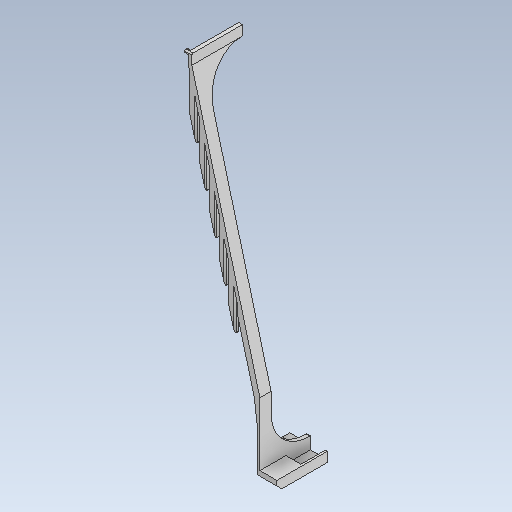
# Autodesk Inventor part: Держатель каскада
Saved by Autodesk Inventor 2020 (Build 240168000, 168)
## iProperties
Created: 2021-05-17
Part Number: Держатель каскада
Material: Типовые
Document SubType Name: Modeling
Designer: I_Love_U_Bogdan
Density: 1 g/cm^3
Appearance: По умолчанию
Author: I_Love_U_Bogdan
Autodesk Inventor part; units mm, degrees
ref_plane "YZ Plane" through (0, 0, 0) normal (1, 0, 0) x (0, 1, 0)
ref_plane "XZ Plane" through (0, 0, 0) normal (0, 1, 0) x (-1, 0, 0)
ref_plane "XY Plane" through (0, 0, 0) normal (0, 0, 1) x (1, 0, 0)
sketch "Эскиз1" plane through (0, 0, 0) normal (0, 0, 1) x (1, 0, 0)
  line L0 (-10.5496, 43.8447) -> (-9.5496, 40.1126)
  line L1 (-9.5496, 26.5897) -> (-9.5496, 40.1126)
  line L2 (-9.5496, 26.5897) -> (-10.5496, 30.3217)
  line L3 (-10.5496, 30.3217) -> (-10.5496, 43.8447)
  line L4 (-6.5496, 28.9165) -> (-5.5496, 25.1844)
  line L5 (-5.5496, 11.6615) -> (-5.5496, 25.1844)
  line L6 (-5.5496, 11.6615) -> (-6.5496, 15.3935)
  line L7 (-6.5496, 15.3935) -> (-6.5496, 28.9165)
  line L8 (-14.5496, 58.7729) -> (-13.5496, 55.0408)
  line L9 (-13.5496, 41.5179) -> (-13.5496, 55.0408)
  line L10 (-13.5496, 41.5179) -> (-14.5496, 45.2499)
  line L11 (-14.5496, 45.2499) -> (-14.5496, 58.7729)
  line L12 (-18.5496, 73.7011) -> (-17.5496, 69.969)
  line L13 (-17.5496, 56.4461) -> (-17.5496, 69.969)
  line L14 (-17.5496, 56.4461) -> (-18.5496, 60.1781)
  line L15 (-18.5496, 60.1781) -> (-18.5496, 73.7011)
  line L16 (-22.5496, 88.6293) -> (-21.5496, 84.8972)
  line L17 (-21.5496, 71.3743) -> (-21.5496, 84.8972)
  line L18 (-21.5496, 71.3743) -> (-22.5496, 75.1063)
  line L19 (-22.5496, 75.1063) -> (-22.5496, 88.6293)
  line L20 (-26.5496, 103.5575) -> (-25.5496, 99.8254)
  line L21 (-25.5496, 86.3025) -> (-25.5496, 99.8254)
  line L22 (-25.5496, 86.3025) -> (-26.5496, 90.0345)
  line L23 (-26.5496, 90.0345) -> (-26.5496, 103.5575)
  line L24 (-5.5496, 31.614) -> (-25.7752, 107.0972)
  line L25 (-25.7752, 110.0635) -> (-25.7752, 107.0972)
  line L26 (-5.5496, 25.1844) -> (-5.5496, 31.614)
  line L27 (-6.5496, 28.9165) -> (-6.5496, 36.5052)
  line L28 (-9.5496, 40.1126) -> (-9.5496, 47.7014)
  line L29 (-10.5496, 43.8447) -> (-10.5496, 51.4334)
  line L30 (-13.5496, 55.0408) -> (-13.5496, 62.6296)
  line L31 (-14.5496, 58.7729) -> (-14.5496, 66.3616)
  line L32 (-17.5496, 69.969) -> (-17.5496, 77.5578)
  line L33 (-18.5496, 73.7011) -> (-18.5496, 81.2898)
  line L34 (-25.5496, 99.8254) -> (-25.5496, 106.2551)
  line L35 (-26.5496, 103.5575) -> (-26.5496, 108.8932)
  line L36 (-21.5496, 84.8972) -> (-21.5496, 91.3269)
  line L37 (-22.5496, 88.6293) -> (-22.5496, 96.218)
  line L38 (-5.5496, 32.7732) -> (-25.7752, 108.2563)
  line L39 (-5.5496, 31.614) -> (-5.5496, 32.7732)
  line L40 (-25.5496, 106.2551) -> (-25.5496, 107.4142)
  line L41 (-21.5496, 84.8972) -> (-21.5496, 92.486)
  line L42 (-5.5496, 17.457) -> (-26.5496, 95.8301)
  line L43 (-28.0432, 111.0635) -> (-27.7752, 110.0635)
  line L44 (-27.7752, 110.0635) -> (-25.7752, 110.0635)
  line L45 (-25.7752, 110.0635) -> (-25.7752, 111.0635)
  line L46 (-25.7752, 111.0635) -> (-28.0432, 111.0635)
  line L47 (-29.7344, 117.3754) -> (-25.7752, 117.3754)
  line L48 (-28.0432, 111.0635) -> (-29.7344, 117.3754)
  line L49 (-25.7752, 111.0635) -> (-28.0432, 111.0635)
  line L50 (-25.7752, 117.3754) -> (-25.7752, 111.0635)
  line L51 (-25.7752, 111.0635) -> (-27.2752, 111.0635)
  line L52 (-27.2752, 111.0635) -> (-27.2752, 112.5635)
  line L53 (-27.2752, 112.5635) -> (-25.7752, 112.5635)
  line L54 (-25.7752, 112.5635) -> (-25.7752, 111.0635)
  line L55 (-25.7752, 112.5635) -> (-24.2752, 112.5635)
  line L56 (-24.2752, 112.5635) -> (-24.2752, 108.4538)
  line L57 (-30.0024, 118.3754) -> (0.8622, 3.1871)
  line L58 (-30.9752, 118.3754) -> (-30.0024, 118.3754)
  line L59 (-30.9752, 108.4603) -> (-30.9752, 118.3754)
  line L60 (-30.4811, 104.7073) -> (-30.9752, 108.4603)
  line L61 (-3.5492, 4.1961) -> (-30.4811, 104.7073)
  line L62 (-3.5492, 4.1961) -> (-3.5492, -15.1653)
  spline S0 degree 3 poles (-3.5492, -15.1653) (-3.5492, -15.4959) (-3.5491, -15.8265) (-3.5502, -16.4901) (-3.5515, -16.823) (-3.5561, -17.1584) knots 0 0 0 0 0.5 0.5 1 1 1 1 weights 1 1 1 1 1 1
  line L63 (-3.5561, -17.1584) -> (2.2248, -22.9393)
  line L64 (2.2248, -7.1624) -> (2.2248, -22.9393)
  line L65 (0.8622, 3.1871) -> (2.2248, -7.1624)
  line L66 (-1.7752, -7.4246) -> (-1.7752, -26.0104)
  line L67 (-1.7752, -26.0104) -> (2.2248, -26.0104)
  line L68 (2.2248, -26.0104) -> (2.2248, -7.1624)
  line L69 (2.2248, -7.1624) -> (0.8622, 3.1871)
  line L70 (0.8622, 3.1871) -> (-4.5492, 23.3829)
  line L71 (-4.5492, 23.3829) -> (-4.5492, 7.9281)
  line L72 (-4.5492, 7.9281) -> (-3.0693, 2.405)
  line L73 (-3.0693, 2.405) -> (-1.7752, -7.4246)
  line L74 (-24.2752, 108.4538) -> (-1.8027, 24.5851)
  line L75 (2.2248, -26.0104) -> (3.7248, -26.0104)
  line L76 (3.7248, -26.0104) -> (3.7248, 3.9564)
  line L77 (3.7248, 3.9564) -> (-1.8027, 24.5851)
  point P0 (0, 0)
  point P1 (-25.5496, 92.098)
  point P2 (-22.5496, 80.9019)
  point P3 (-21.5496, 77.1698)
  point P4 (-18.5496, 65.9737)
  point P5 (-17.5496, 62.2416)
  point P6 (-14.5496, 51.0455)
  point P7 (-13.5496, 47.3134)
  point P8 (-10.5496, 36.1173)
  point P9 (-9.5496, 32.3852)
  point P10 (-6.5496, 21.1891)
  point P11 (-5.5496, 27.1163)
  dimension "d0" = 0.3
  dimension "d1" = 2
  dimension "d2" = 1.5
  dimension "d3" = 1.5
  dimension "d4" = 1.5
  dimension "d6" = 1.5
  dimension "d7" = 2.9641
  dimension "d8" = 1.5
  constraints: 80 end point, 13 vertical, 8 parallel, 7 point on line, 3 horizontal, 2 perpendicular, 16 other
  measures "d1" distance between parallel lines of L12 L42
  measures "d2" distance of L51.end L52.end
  measures "d3" distance of L52.end L53.end
  measures "d4" distance of L53.end L55.end
  measures "d7" distance between parallel lines of L77 L57
  measures "d8" distance between parallel lines of L76 L64
extrude "Выдавливание1" add sketch "Эскиз1" against normal blind 1.6 contours L3 L42 L9 L30 L57 L29 | L28 L57 L27 L7 L42 L1 | L57 L30 L24 L29 | L28 L24 L27 L57 | L24 L30 L38 L29 | L28 L38 L27 L24 | L42 L13 L32 L57 L31 L11 | L38 L25 L45 L50 L55 L56 L74 L77 L76 L75 L68 L64 L65 L57 L26 L39 | L57 L32 L24 L31 | L24 L32 L38 L31 | L42 L17 L36 L57 L33 L15 | L57 L36 L24 L33 | L24 L41 L38 L33 | L42 L21 L34 L57 L37 L19 | L57 L34 L24 L37 | L24 L40 L38 L37 | L52 L53 L50 L46
sketch "Эскиз2" plane through (0, 0, -1.6) normal (0, 0, -1) x (-1, 0, 0)
  line L0 (-3.7248, -26.0104) -> (-2.2248, -26.0104) projected
  line L1 (-2.2248, -26.0104) -> (-2.2248, -7.1624) projected
  line L2 (-2.2248, -7.1624) -> (-0.8622, 3.1871) projected
  line L3 (-0.8622, 3.1871) -> (5.5496, 27.1163) projected
  line L4 (5.5496, 27.1163) -> (5.5496, 32.7732) projected
  line L5 (5.5496, 32.7732) -> (6.5496, 36.5052) projected
  line L6 (6.5496, 36.5052) -> (6.5496, 21.1891) projected
  line L7 (6.5496, 21.1891) -> (9.5496, 32.3852) projected
  line L8 (9.5496, 32.3852) -> (9.5496, 47.7014) projected
  line L9 (9.5496, 47.7014) -> (10.5496, 51.4334) projected
  line L10 (10.5496, 51.4334) -> (10.5496, 36.1173) projected
  line L11 (10.5496, 36.1173) -> (13.5496, 47.3134) projected
  line L12 (13.5496, 47.3134) -> (13.5496, 62.6296) projected
  line L13 (13.5496, 62.6296) -> (14.5496, 66.3616) projected
  line L14 (14.5496, 66.3616) -> (14.5496, 51.0455) projected
  line L15 (14.5496, 51.0455) -> (17.5496, 62.2416) projected
  line L16 (17.5496, 62.2416) -> (17.5496, 77.5578) projected
  line L17 (17.5496, 77.5578) -> (18.5496, 81.2898) projected
  line L18 (18.5496, 81.2898) -> (18.5496, 65.9737) projected
  line L19 (18.5496, 65.9737) -> (21.5496, 77.1698) projected
  line L20 (21.5496, 77.1698) -> (21.5496, 92.486) projected
  line L21 (21.5496, 92.486) -> (22.5496, 96.218) projected
  line L22 (22.5496, 96.218) -> (22.5496, 80.9019) projected
  line L23 (22.5496, 80.9019) -> (25.5496, 92.098) projected
  line L24 (25.5496, 92.098) -> (25.5496, 107.4142) projected
  line L25 (25.5496, 107.4142) -> (25.7752, 108.2563) projected
  line L26 (25.7752, 108.2563) -> (25.7752, 111.0635) projected
  line L27 (25.7752, 111.0635) -> (27.2752, 111.0635) projected
  line L28 (27.2752, 111.0635) -> (27.2752, 112.5635) projected
  line L29 (27.2752, 112.5635) -> (24.2752, 112.5635) projected
  line L30 (24.2752, 112.5635) -> (24.2752, 108.4538) projected
  line L31 (24.2752, 108.4538) -> (-3.7248, 3.9564) projected
  line L32 (-3.7248, 3.9564) -> (-3.7248, -26.0104) projected
  line L33 (25.5496, 107.4142) -> (-2.2248, 3.7589)
  line L34 (-2.2248, -26.0104) -> (-2.2248, -7.1624) projected
  line L35 (-2.2248, -7.1624) -> (-2.2248, 3.7589)
  line L36 (25.7752, 111.0635) -> (25.7752, 112.5635)
  line L37 (27.2752, 112.5635) -> (24.2752, 112.5635) projected
  point P0 (0, 0)
  dimension "d11" = 1.5
  constraints: 6 end point, 1 collinear, 1 midpoint, 1 parallel, 1 point on line
  measures "d11" distance between parallel lines of L31 L33
extrude "Выдавливание2" add sketch "Эскиз2" along normal blind 3 contours L32 L31 L30 L29 L36 L26 L25 L33 L21 L17 L13 L9 L5 L35 L1 L0
chamfer "Фаска1" distance 0.5 angle 45 25 edges at (-6.5496, 21.1891, -0.8) (-9.5496, 32.3852, -0.8) (-10.5496, 36.1173, -0.8) (-13.5496, 47.3134, -0.8) (-14.5496, 51.0455, -0.8) (-17.5496, 62.2416, -0.8) (-18.5496, 65.9737, -0.8) (-21.5496, 77.1698, -0.8) (-22.5496, 80.9019, -0.8) (-25.5496, 92.098, -0.8) (-26.5252, 111.0635, 0) (-25.7752, 112.5635, 0) (-6.5496, 28.8471, 0) (-9.5496, 40.0433, 0) (-10.5496, 43.7753, 0) (-13.5496, 54.9715, 0) (-14.5496, 58.7035, 0) (-17.5496, 69.8997, 0) (-18.5496, 73.6317, 0) (-21.5496, 84.8279, 0) (-22.5496, 88.5599, 0) (-25.5496, 99.7561, 0) (-2.3437, 15.1517, 0) (1.5435, -1.9877, 0) (2.2248, -16.5864, 0)
sketch "Эскиз3" plane through (0, 0, -4.6) normal (0, 0, -1) x (-1, 0, 0)
  line L0 (-2.7248, -26.0104) -> (-2.7248, -7.1296) projected
  line L1 (-2.2248, 3.7589) -> (25.7752, 108.2563) projected
  line L2 (25.7752, 108.2563) -> (25.7752, 112.5635) projected
  line L3 (25.7752, 112.5635) -> (24.2752, 112.5635) projected
  line L4 (24.2752, 112.5635) -> (24.2752, 108.4538) projected
  line L5 (24.2752, 108.4538) -> (-3.7248, 3.9564) projected
  line L6 (-3.7248, 3.9564) -> (-3.7248, -26.0104) projected
  line L7 (-3.7248, -26.0104) -> (-2.2248, -26.0104) projected
  line L8 (-2.2248, -26.0104) -> (-2.2248, 3.7589) projected
  line L9 (-3.7248, 3.9564) -> (-3.7248, -26.0104) projected
  line L10 (-2.2248, -26.0104) -> (-3.7248, -26.0104)
  line L11 (-3.7248, -26.0104) -> (-3.7248, -20.0104)
  line L12 (-3.7248, -20.0104) -> (-2.2248, -20.0104)
  line L13 (-2.2248, -20.0104) -> (-2.2248, -26.0104)
  line L14 (25.7752, 112.5635) -> (24.2752, 112.5635) projected
  line L15 (24.2752, 112.5635) -> (24.2752, 108.4538) projected
  line L16 (25.7752, 112.5635) -> (24.2752, 112.5635)
  line L17 (24.2752, 112.5635) -> (24.2752, 108.4538)
  line L18 (24.2752, 108.4538) -> (25.7752, 108.4538)
  line L19 (25.7752, 108.4538) -> (25.7752, 112.5635)
  point P0 (0, 0)
  dimension "d17" = 6
  constraints: 16 end point, 4 parallel, 2 horizontal, 2 perpendicular, 1 point on line
  measures "d17" distance between parallel lines of L7 L12
extrude "Выдавливание3" add sketch "Эскиз3" along normal blind 16.2 contours L7 L6 L12 L0 | L0 L12 L8 L7 | L4 L3 L2 L18
sketch "Эскиз4" plane through (2.2248, -7.1624, -1.6) normal (-1, 0, 0) x (0, 0, 1)
  arc A0 (-16.2, -18.8053) -> (-16.2, -15.8053) centre (-16.2, -17.3053) ccw projected
  line L0 (-16.2, -15.8053) -> (-22.2, -15.8053) projected
  line L1 (1.1, 0) -> (1.1, -18.848) projected
  line L2 (1.1, 0) -> (0, 0) projected
  line L3 (0, 10.9213) -> (0, 0) projected
  line L4 (0, 10.9213) -> (-3, 10.9213) projected
  line L5 (-3, -12.848) -> (-3, 10.9213) projected
  line L6 (-3, -12.848) -> (-19.2, -12.848) projected
  line L7 (-19.2, -18.848) -> (-19.2, -12.848) projected
  line L8 (1.1, -18.848) -> (-19.2, -18.848) projected
  arc A1 (-16.2, -18.6053) -> (-16.2, -16.0053) centre (-16.2, -17.3053) ccw
  line L9 (-16.2, -16.0053) -> (-19.2, -16.0053)
  line L10 (-16.2, -18.6053) -> (-19.2, -18.6053)
  point P0 (1.6, 7.1624)
  dimension "d20" = 0.2
  constraints: 4 end point, 2 point on circle, 2 point on line, 1 centre point, 1 horizontal
  measures "d20" radial gap between concentric circles of A0 A1
extrude "Выдавливание4" add sketch "Эскиз4" along normal blind 7 contours L7 L9 A1 L10
sketch "Эскиз5" plane through (3.7248, -26.0104, 0) normal (1, 0, 0) x (0, 0, -1)
  line L0 (20.8, 6) -> (20.8, 0) projected
  line L1 (0, 0) -> (20.8, 0)
  line L2 (20.8, 0) -> (20.8, 4)
  line L3 (20.8, 4) -> (0, 4)
  line L4 (0, 4) -> (0, 0)
  point P0 (0, 26.0104)
  dimension "d23" = 4
  constraints: 8 end point, 2 parallel, 1 horizontal, 1 perpendicular, 1 point on line
  measures "d23" distance between parallel lines of L1 L3
extrude "Выдавливание5" add sketch "Эскиз5" along normal blind 7
sketch "Эскиз6" plane through (3.7248, -22.0104, 0) normal (0, 1, 0) x (1, 0, 0)
  line L0 (0, 4.6) -> (0, 20.8) projected
  line L1 (0, 20.8) -> (7, 20.8) projected
  line L2 (0, 10.7) -> (6.2, 10.7)
  line L3 (6.2, 10.7) -> (6.2, 20.8)
  line L4 (6.2, 20.8) -> (0, 20.8)
  line L5 (0, 20.8) -> (0, 10.7)
  point P0 (-3.7248, 0)
  dimension "d26" = 10.1
  dimension "d27" = 6.2
  constraints: 8 end point, 2 parallel, 2 point on line, 1 horizontal, 1 perpendicular
  measures "d26" distance of L2.end L3.end
  measures "d27" distance of L2.start L2.end
extrude "Выдавливание6" cut sketch "Эскиз6" against normal blind 3
fillet "Сопряжение1" radius 16 2 edges at (2.9748, -20.0104, -4.6) (-25.0252, 108.4538, -4.6)
chamfer "Фаска2" distance 2 angle 45 1 edges at (6.7248, -26.0104, 0)
fillet "Сопряжение2" radius 0.7 2 edges at (-26.5252, 111.0635, -1.6) (-26.5252, 112.5635, -1.6)
